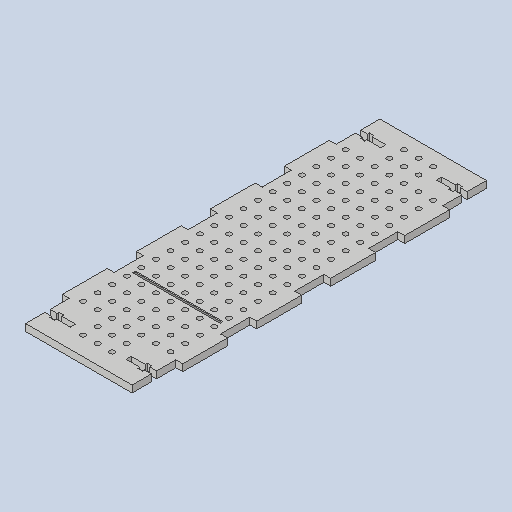
# Autodesk Inventor part: V3 Mounting Plate
Saved by Autodesk Inventor 2022.1 (Build 261234020, 234B)
## iProperties
Created: 2020-05-07
Part Number: V3 Mounting Plate
Material: Generic
Document SubType Name: Modeling
Designer: Workshop Tech
Density: 1 g/cm^3
Appearance: Default
Author: Workshop Tech
Autodesk Inventor part; units mm, degrees
ref_plane "YZ Plane" through (0, 0, 0) normal (1, 0, 0) x (0, 1, 0)
ref_plane "XZ Plane" through (0, 0, 0) normal (0, 1, 0) x (-1, 0, 0)
ref_plane "XY Plane" through (0, 0, 0) normal (0, 0, 1) x (1, 0, 0)
sketch "Sketch1" plane through (0, 0, 0) normal (0, 1, 0) x (-1, 0, 0)
  line L0 (0, 0) -> (104.71, 0)
  line L1 (104.71, 0) -> (104.71, -308.4068)
  line L2 (104.71, -308.4068) -> (0, -308.4068)
  line L3 (0, -308.4068) -> (0, 0)
  dimension "d0" = 104.71
  dimension "d1" = 308.4068
  constraints: 8 end point, 2 parallel, 1 horizontal, 1 perpendicular
  measures "d0" distance between parallel lines of L3 L1
  measures "d1" distance between parallel lines of L2 L0
extrude "Base" add sketch "Sketch1" along normal blind 6
sketch "Sketch7" plane through (0, 6, 0) normal (0, 1, 0) x (1, 0, 0)
  line L0 (0, 0) -> (0, 308.4068) projected
  line L1 (-104.71, 0) -> (0, 0) projected
  line L2 (-104.71, 0) -> (0, 0) projected
  line L3 (0, 0) -> (0, 308.4068) projected
  line L4 (0, 308.4068) -> (-104.71, 308.4068) projected
  line L5 (-104.71, 308.4068) -> (-104.71, 0) projected
  point P0 (-52.355, 270.3068)
  dimension "d35" = 38.1
  dimension "d36" = 52.355
  measures "d35" distance from line of L4 point (-52.355, 270.307)
  measures "d36" distance from line of L5 point (-52.355, 270.307)
hole "Board Hole" at (-52.355, 6, -270.3068) direction (0, -1, 0) diameter 4.5 end through all clearance for "Flat Head Machine Screw" size "M4" standard "Ansi Metric M Profile"
pattern_linear "Patterned Board Holes" count 19 spacing 12.7 along (0, 0, 1) count 7 spacing 12.7 along (1, 0, 0) of "Board Hole" second direction both ways yes
sketch "Sketch12" plane through (0, 6, 0) normal (0, 1, 0) x (1, 0, 0)
  line L0 (0, 308.4068) -> (0, 0) projected
  line L1 (-104.71, 0) -> (-104.71, 308.4068) projected
  line L2 (0, 0) -> (-6, 0)
  line L3 (-6, 0) -> (-6, 38.1)
  line L4 (-6, 38.1) -> (0, 38.1)
  line L5 (0, 38.1) -> (0, 0)
  line L6 (-104.71, 0) -> (0, 0) projected
  line L7 (-104.71, 0) -> (-98.71, 0)
  line L8 (-98.71, 0) -> (-98.71, 38.1)
  line L9 (-98.71, 38.1) -> (-104.71, 38.1)
  line L10 (-104.71, 38.1) -> (-104.71, 0)
  dimension "d188" = 6
  dimension "d189" = 38.1
  dimension "d190" = 6
  dimension "d191" = 38.1
  constraints: 16 end point, 4 parallel, 2 horizontal, 2 perpendicular
  measures "d188" distance of L3.end L4.end
  measures "d189" distance of L2.end L3.end
  measures "d190" distance of L9.end L8.end
  measures "d191" distance of L8.end L7.end
extrude "Extrusion4" cut sketch "Sketch12" against normal blind 25.4
sketch "Sketch13" plane through (0, 6, 0) normal (0, 1, 0) x (1, 0, 0)
  line L0 (0, 0) -> (0, 308.4068) projected
  line L1 (0, 308.4068) -> (-6, 308.4068)
  line L2 (-6, 270.3068) -> (0, 270.3068)
  line L3 (-6, 270.3068) -> (-6, 308.4068)
  line L4 (0, 308.4068) -> (0, 0) projected
  line L5 (0, 270.3068) -> (0, 308.4068)
  line L6 (0, 308.4068) -> (-104.71, 308.4068) projected
  line L7 (-104.71, 308.4068) -> (-98.71, 308.4068)
  line L8 (-98.71, 308.4068) -> (-98.71, 270.3068)
  line L9 (-98.71, 270.3068) -> (-104.71, 270.3068)
  line L10 (-104.71, 270.3068) -> (-104.71, 308.4068)
  point P0 (0, 38.1)
  point P1 (0, 270.3068)
  dimension "d175" = 38.1
  dimension "d176" = 6
  dimension "d177" = 6
  dimension "d178" = 6
  dimension "d179" = 38.1
  constraints: 16 end point, 2 horizontal, 2 parallel, 1 collinear, 1 perpendicular, 1 vertical
  measures "d175" distance of L2.start L1.end
  measures "d176" distance of L2.start L2.end
  measures "d177" distance of L0.end L1.end
  measures "d178" distance of L8.end L9.end
  measures "d179" distance of L7.end L8.end
sketch "Sketch16" plane through (0, 6, 0) normal (0, 1, 0) x (1, 0, 0)
  circle A0 centre (-52.355, 270.3068) radius 2.25 projected
  point P0 (0, 0)
  point P1 (-52.355, 283.0068)
  dimension "d163" = 12.7
  measures "d163" distance of A0.centre point (-52.355, 283.007)
hole "Hole9" at (-52.355, 6, -283.0068) direction (0, -1, 0) diameter 4.5 end through all clearance for "Flat Head Machine Screw" size "M4" standard "Ansi Metric M Profile"
sketch "Sketch17" plane through (0, 6, 0) normal (0, 1, 0) x (1, 0, 0)
  line L0 (-104.71, 141.5034) -> (-98.71, 141.5034)
  line L1 (-98.71, 141.5034) -> (-98.71, 166.9034)
  line L2 (-98.71, 166.9034) -> (-104.71, 166.9034)
  line L3 (-104.71, 166.9034) -> (-104.71, 141.5034)
  line L4 (-104.71, 77.1017) -> (-98.71, 77.1017)
  line L5 (-98.71, 77.1017) -> (-98.71, 102.5017)
  line L6 (-98.71, 102.5017) -> (-104.71, 102.5017)
  line L7 (-104.71, 102.5017) -> (-104.71, 77.1017)
  line L8 (-104.71, 205.9051) -> (-98.71, 205.9051)
  line L9 (-98.71, 205.9051) -> (-98.71, 231.3051)
  line L10 (-98.71, 231.3051) -> (-104.71, 231.3051)
  line L11 (-104.71, 231.3051) -> (-104.71, 205.9051)
  line L12 (-6, 77.1017) -> (0, 77.1017)
  line L13 (0, 77.1017) -> (0, 102.5017)
  line L14 (0, 102.5017) -> (-6, 102.5017)
  line L15 (-6, 102.5017) -> (-6, 77.1017)
  line L16 (-6, 141.5034) -> (0, 141.5034)
  line L17 (0, 141.5034) -> (0, 166.9034)
  line L18 (0, 166.9034) -> (-6, 166.9034)
  line L19 (-6, 166.9034) -> (-6, 141.5034)
  line L20 (-6, 205.9051) -> (0, 205.9051)
  line L21 (0, 205.9051) -> (0, 231.3051)
  line L22 (0, 231.3051) -> (-6, 231.3051)
  line L23 (-6, 231.3051) -> (-6, 205.9051)
  line L24 (-104.71, 308.4068) -> (-104.71, 38.1) projected
  line L25 (0, 38.1) -> (0, 308.4068) projected
  line L26 (-98.71, 0) -> (-6, 0) projected
  line L27 (0, 308.4068) -> (-104.71, 308.4068) projected
  line L28 (-52.355, 0) -> (-52.355, 308.4068)
  point P0 (-6, 154.2034)
  point P1 (-98.71, 154.2034)
  point P2 (-52.355, 154.2034)
  dimension "d193" = 6
  dimension "d194" = 25.4
  dimension "d195" = 6
  dimension "d196" = 25.4
  dimension "d197" = 6
  dimension "d198" = 25.4
  dimension "d199" = 6
  dimension "d200" = 6
  dimension "d201" = 6
  dimension "d202" = 39.0017
  dimension "d203" = 39.0017
  dimension "d204" = 39.0017
  dimension "d205" = 39.0017
  dimension "d206" = 25.4
  dimension "d207" = 25.4
  dimension "d208" = 25.4
  constraints: 50 end point, 12 parallel, 6 horizontal, 6 perpendicular, 6 point on line, 5 midpoint, 2 horizontal alignment
  measures "d193" distance of L2.end L1.end
  measures "d194" distance of L1.end L0.end
  measures "d195" distance of L6.end L5.end
  measures "d196" distance of L5.end L4.end
  measures "d197" distance of L10.end L9.end
  measures "d198" distance of L9.end L8.end
  measures "d199" distance of L14.end L13.end
  measures "d200" distance of L18.end L17.end
  measures "d201" distance of L22.end L21.end
  measures "d202" distance between parallel lines of L16 L14
  measures "d203" distance from line of L20.start L18
  measures "d204" vertical distance of L1.end L8.start
  measures "d205" distance between parallel lines of L6 L0
  measures "d206" distance of L22.end L20.start
  measures "d207" distance of L18.end L16.start
  measures "d208" distance of L14.end L12.start
extrude "Extrusion6" cut sketch "Sketch17" against normal blind 25.4
extrude "Extrusion7" cut sketch "Sketch13" against normal blind 25.4
sketch "Sketch18" plane through (0, 6, 0) normal (0, 1, 0) x (1, 0, 0)
  line L0 (-52.355, 0) -> (-52.355, 308.4068)
  line L1 (-133.0597, 154.2034) -> (31.0499, 154.2034)
  line L2 (0, 291.6047) -> (0, 287.1089) projected
  line L3 (0, 291.6047) -> (0, 287.1089) projected
  line L4 (-28, 287.1089) -> (-28, 291.6047)
  line L5 (0, 291.6047) -> (0, 287.1089)
  line L6 (-16, 285.3568) -> (-12, 285.3568)
  line L7 (-12, 293.3568) -> (-16, 293.3568)
  line L8 (0, 287.1089) -> (-12, 287.1089)
  line L9 (-16, 287.1089) -> (-28, 287.1089)
  line L10 (-28, 291.6047) -> (-16, 291.6047)
  line L11 (-12, 291.6047) -> (0, 291.6047)
  line L12 (-16, 293.3568) -> (-16, 291.6047)
  line L13 (-16, 287.1089) -> (-16, 285.3568)
  line L14 (-12, 285.3568) -> (-12, 287.1089)
  line L15 (-12, 291.6047) -> (-12, 293.3568)
  line L16 (28.3497, 154.2034) -> (-135.7599, 154.2034)
  line L17 (-104.71, 291.6047) -> (-104.71, 287.1089)
  line L18 (-76.71, 287.1089) -> (-76.71, 291.6047)
  line L19 (-88.71, 285.3568) -> (-92.71, 285.3568)
  line L20 (-92.71, 293.3568) -> (-88.71, 293.3568)
  line L21 (-104.71, 287.1089) -> (-92.71, 287.1089)
  line L22 (-88.71, 287.1089) -> (-76.71, 287.1089)
  line L23 (-76.71, 291.6047) -> (-88.71, 291.6047)
  line L24 (-92.71, 291.6047) -> (-104.71, 291.6047)
  line L25 (-88.71, 293.3568) -> (-88.71, 291.6047)
  line L26 (-88.71, 287.1089) -> (-88.71, 285.3568)
  line L27 (-92.71, 285.3568) -> (-92.71, 287.1089)
  line L28 (-92.71, 291.6047) -> (-92.71, 293.3568)
  line L29 (0, 16.8021) -> (0, 21.2979)
  line L30 (-28, 21.2979) -> (-28, 16.8021)
  line L31 (-16, 23.05) -> (-12, 23.05)
  line L32 (-12, 15.05) -> (-16, 15.05)
  line L33 (0, 21.2979) -> (-12, 21.2979)
  line L34 (-16, 21.2979) -> (-28, 21.2979)
  line L35 (-28, 16.8021) -> (-16, 16.8021)
  line L36 (-12, 16.8021) -> (0, 16.8021)
  line L37 (-16, 15.05) -> (-16, 16.8021)
  line L38 (-16, 21.2979) -> (-16, 23.05)
  line L39 (-12, 23.05) -> (-12, 21.2979)
  line L40 (-12, 16.8021) -> (-12, 15.05)
  line L41 (-104.71, 21.2979) -> (-92.71, 21.2979)
  line L42 (-104.71, 16.8021) -> (-104.71, 21.2979)
  line L43 (-92.71, 16.8021) -> (-104.71, 16.8021)
  line L44 (-92.71, 16.8021) -> (-92.71, 15.05)
  line L45 (-92.71, 15.05) -> (-88.71, 15.05)
  line L46 (-88.71, 15.05) -> (-88.71, 16.8021)
  line L47 (-76.71, 16.8021) -> (-88.71, 16.8021)
  line L48 (-76.71, 21.2979) -> (-76.71, 16.8021)
  line L49 (-88.71, 21.2979) -> (-76.71, 21.2979)
  line L50 (-88.71, 21.2979) -> (-88.71, 23.05)
  line L51 (-88.71, 23.05) -> (-92.71, 23.05)
  line L52 (-92.71, 23.05) -> (-92.71, 21.2979)
  line L53 (-6, 308.4068) -> (-98.71, 308.4068) projected
  point P0 (0, 0)
  point P1 (-6, 270.3068)
  point P2 (-98.71, 0)
  point P3 (-19.9732, 289.3568)
  point P4 (0, 289.3568)
  point P5 (0, 289.3568)
  dimension "d237" = 28
  dimension "d238" = 4
  dimension "d239" = 8
  dimension "d240" = 12
  dimension "d242" = 16.8021
  constraints: 102 end point, 41 symmetric about line, 10 parallel, 4 horizontal, 4 perpendicular, 3 midpoint, 2 equal length, 1 horizontal alignment
  measures "d237" distance of L4.end L5.start
  measures "d238" distance of L7.end L7.start
  measures "d239" distance of L7.start L6.end
  measures "d240" distance of L11.start L5.start
  measures "d242" distance between parallel lines of L53 L11
extrude "Extrusion8" cut sketch "Sketch18" against normal blind 25.4
pattern_linear "Rectangular Pattern6" count 2 spacing 12.7 along (0, 0, -1) count 3 spacing 12.7 along (-1, 0, 0) of "Hole9" second direction both ways yes
sketch "Sketch19" plane through (0, 6, 0) normal (0, 1, 0) x (1, 0, 0)
  circle A0 centre (-52.355, 29.0068) radius 1.6256
  point P0 (0, 0)
  dimension "d225" = 3.2512
  constraints: 1 centre point
  measures "d225" diameter of A0
sketch "Sketch20" plane through (0, 6, 0) normal (0, 1, 0) x (1, 0, 0)
  line L0 (-14.255, 87.4268) -> (-90.455, 87.4268)
  line L1 (-90.455, 87.4268) -> (-90.455, 84.8868)
  line L2 (-90.455, 84.8868) -> (-14.255, 84.8868)
  line L3 (-14.255, 84.8868) -> (-14.255, 87.4268)
  point P0 (0, 0)
  dimension "d234" = 2.54
  constraints: 8 end point, 2 parallel, 1 horizontal, 1 perpendicular
  measures "d234" distance of L1.end L0.end
extrude "Extrusion10" cut sketch "Sketch20" against normal blind 1
hole "Hole10" at (-52.355, 6, -29.0068) direction (0, -1, 0) diameter 4.5 end through all clearance for "Flat Head Machine Screw" size "M4" standard "Ansi Metric M Profile"
pattern_linear "Rectangular Pattern8" count 3 spacing 12.7 along (1, 0, 0) count 2 spacing 12.7 along (0, 0, 1) of "Hole10" first direction both ways yes
body "Solid1"
